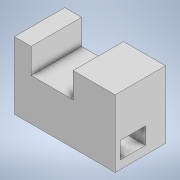
# Autodesk Inventor part: 4.2 Part B
Saved by Autodesk Inventor 2020 (Build 240168000, 168)
## iProperties
Created: 2020-01-07
Part Number: 4.2 Part B
Material: Generic
Document SubType Name: Modeling
Designer: cks4a449
Density: 1 g/cm^3
Appearance: Default
Author: cks4a449
Autodesk Inventor part; units mm, degrees
ref_plane "YZ Plane" through (0, 0, 0) normal (1, 0, 0) x (0, 1, 0)
ref_plane "XZ Plane" through (0, 0, 0) normal (0, 1, 0) x (-1, 0, 0)
ref_plane "XY Plane" through (0, 0, 0) normal (0, 0, 1) x (1, 0, 0)
sketch "Sketch1" plane through (0, 0, 0) normal (0, 0, 1) x (1, 0, 0)
  line L0 (0, 0) -> (60, 0)
  line L1 (0, 0) -> (0, 40)
  line L2 (0, 40) -> (10, 40)
  line L3 (10, 40) -> (10, 25)
  line L4 (10, 25) -> (35, 25)
  line L5 (35, 25) -> (35, 40)
  line L6 (35, 40) -> (60, 40)
  line L7 (60, 40) -> (60, 0)
  dimension "d0" = 60
  dimension "d1" = 40
  dimension "d2" = 10
  dimension "d3" = 15
  dimension "d4" = 25
  dimension "d5" = 15
  dimension "d6" = 25
  constraints: 16 end point, 3 perpendicular, 2 point on line, 1 horizontal, 1 vertical
  measures "d0" distance of L0.start L0.end
  measures "d1" distance of L0.start L1.end
  measures "d2" distance of L1.end L2.end
  measures "d3" distance of L2.end L3.end
  measures "d4" distance of L3.end L4.end
  measures "d5" distance of L4.end L5.end
  measures "d6" distance of L5.end L6.end
extrude "Extrusion1" add sketch "Sketch1" along normal blind 30
sketch "Sketch2" plane through (60, 0, 0) normal (1, 0, 0) x (0, 0, -1)
  line L0 (-30, 40) -> (-30, 0) projected
  line L1 (-30, 0) -> (-27, 0)
  line L2 (-30, 5) -> (-30, 0)
  line L3 (-27, 5) -> (-12, 5)
  line L4 (-12, 5) -> (-12, 15)
  line L5 (-12, 15) -> (-27, 15)
  line L6 (-27, 15) -> (-27, 5)
  point P0 (0, 0)
  dimension "d9" = 3
  dimension "d10" = 5
  dimension "d11" = 15
  dimension "d12" = 10
  constraints: 12 end point, 2 horizontal, 2 parallel, 1 perpendicular
  measures "d9" distance of L2.start L3.start
  measures "d10" distance of L3.start L1.end
  measures "d11" distance of L5.end L4.end
  measures "d12" distance of L4.end L3.end
extrude "Extrusion2" cut sketch "Sketch2" against normal up to surface (60 mm away)
body "Solid1"
